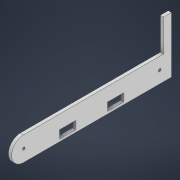
# Autodesk Inventor part: Стенка конвейера
Saved by Autodesk Inventor 2022 (Build 260153000, 153)
## iProperties
Created: 2023-02-18
Part Number: Стенка конвейера
Material: Типовые
Document SubType Name: Modeling
Designer: Глеб
Density: 1 g/cm^3
Appearance: По умолчанию
Author: Глеб
Autodesk Inventor part; units mm, degrees
ref_plane "YZ Plane" through (0, 0, 0) normal (1, 0, 0) x (0, 1, 0)
ref_plane "XZ Plane" through (0, 0, 0) normal (0, 1, 0) x (-1, 0, 0)
ref_plane "XY Plane" through (0, 0, 0) normal (0, 0, 1) x (1, 0, 0)
sketch "Эскиз1" plane through (0, 0, 0) normal (1, 0, 0) x (0, 1, 0)
  line L0 (0, 100) -> (0, -100)
  line L1 (0, -100) -> (30, -100)
  line L2 (30, -100) -> (30, 100)
  line L3 (30, 100) -> (0, 100)
  line L4 (-14, 0) -> (84, 0) construction
  line L5 (0, -140) -> (0, 140) construction
  line L6 (30, -100) -> (70, -100)
  line L7 (70, -100) -> (70, -90)
  line L8 (70, -90) -> (30, -90)
  line L9 (30, -90) -> (30, -100)
  point P0 (0, 0)
  dimension "d0" = 200
  dimension "d1" = 30
  dimension "d2" = 10
  dimension "d3" = 40
  constraints: 16 end point, 4 parallel, 2 perpendicular, 1 midpoint, 1 point on line, 1 vertical, 1 other
  measures "d0" distance between parallel lines of L3 L1
  measures "d1" distance between parallel lines of L0 L2
  measures "d2" distance of L6.end L7.end
  measures "d3" distance between parallel lines of L2 L7
extrude "Выдавливание1" add sketch "Эскиз1" along normal mid plane 4
fillet "Сопряжение1" radius 15 2 edges at (0, 30, 100) (0, 0, 100)
sketch "Эскиз2" plane through (2, 0, 0) normal (1, 0, 0) x (0, 0, -1)
  line L0 (-20, 13) -> (-40, 13)
  line L1 (-85, 0) -> (100, 0) construction
  line L2 (100, 0) -> (100, 70) projected
  line L3 (-40, 13) -> (-20, 13)
  line L4 (-20, 13) -> (-20, 3)
  line L5 (-20, 3) -> (-40, 3)
  line L6 (-40, 3) -> (-40, 13)
  line L7 (20, 13) -> (40, 13)
  line L8 (40, 13) -> (40, 3)
  line L9 (40, 3) -> (20, 3)
  line L10 (20, 3) -> (20, 13)
  point P0 (0, 0)
  point P1 (57.0517, 0.6179)
  dimension "d26" = 10
  dimension "d27" = 20
  dimension "d28" = 3
  dimension "d29" = 20
  dimension "d31" = 20
  dimension "d34" = 3
  dimension "d35" = 10
  dimension "d36" = 20
  constraints: 18 end point, 4 parallel, 2 horizontal, 2 perpendicular
  measures "d26" distance between parallel lines of L0 L5
  measures "d27" distance between parallel lines of L4 L6
  measures "d28" distance between parallel lines of L1 L5
  measures "d29" distance from line of point (0, 0) L4
  measures "d31" distance between parallel lines of L8 L10
  measures "d34" distance between parallel lines of L1 L9
  measures "d35" distance of L9.end L7.start
  measures "d36" distance from line of point (0, 0) L10
extrude "Выдавливание2" cut sketch "Эскиз2" against normal blind 4
sketch "Эскиз3" plane through (2, 0, 0) normal (1, 0, 0) x (0, 0, -1)
  arc A0 (-85, 30) -> (-85, 0) centre (-85, 15) ccw projected
  line L0 (90, 30) -> (-85, 30) projected
  line L1 (100, 0) -> (100, 70) projected
  point P0 (0, 0)
  point P1 (85, 15)
  dimension "d16" = 15
  dimension "d17" = 15
  constraints: 1 coincident
  measures "d16" distance from line of L0 point (85, 15)
  measures "d17" distance from line of L1 point (85, 15)
hole "Отверстие1" at (2, 15, -85) at (2, 15, 85) direction (-1, 0, 0) diameter 3 depth 4
fillet "Сопряжение2" radius 0.1 4 edges at (2, 15, -83.5) (2, 15, 86.5) (-2, 15, -83.5) (-2, 15, 86.5)
